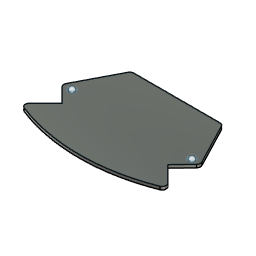
moter-size (Autodesk Fusion 360 design; units mm, degrees)
Autodesk Fusion 360 part; units mm, degrees
sketch "スケッチ1" plane through (0, 0, 0) normal (0, 0, 1) x (1, 0, 0)
  arc A0 (-42.8671, 10.2928) -> (42.0947, 10.2928) centre (-0.3862, 91.8977) ccw
  line L0 (-0.3862, 91.8977) -> (-42.8671, 10.2928) construction
  line L1 (-0.3862, 91.8977) -> (42.0947, 10.2928) construction
  line L2 (-42.8671, 10.2928) -> (-23.0119, 48.4342)
  line L3 (42.0947, 10.2928) -> (22.2395, 48.4342)
  line L4 (-23.0119, 48.4342) -> (22.2395, 48.4342)
  dimension "d1" = 92
  dimension "d2" = 55
  dimension "d3" = 43
  dimension "d4" = 43
  constraint parallel L0 L2
  constraint parallel L1 L3
  measures "d1" radius of A0
  measures "d2" angle of L0 L1
  measures "d3" distance of A0.start L2.end
  measures "d4" distance of A0.end L3.end
extrude "押し出し1" add sketch "スケッチ1" along normal blind 1.5
sketch "スケッチ2" plane through (0, 0, 1.5) normal (0, 0, 1) x (-1, 0, 0)
  arc A0 (42.8671, -10.2928) -> (-42.0947, -10.2928) centre (0.3862, -91.8977) ccw
  line L0 (-42.0947, -10.2928) -> (-22.2395, -48.4342)
  line L1 (-22.2395, -48.4342) -> (23.0119, -48.4342)
  line L2 (23.0119, -48.4342) -> (42.8671, -10.2928)
  line L3 (42.8671, -10.2928) -> (34.7865, -25.8154)
  line L4 (-42.0947, -10.2928) -> (-34.0141, -25.8154)
  line L5 (34.7865, -25.8154) -> (26.6537, -17.6847)
  line L6 (26.6537, -17.6847) -> (36.8874, -7.4486)
  line L7 (36.8874, -7.4486) -> (42.8671, -10.2928)
  line L8 (34.7865, -25.8154) -> (42.8671, -10.2928)
  line L9 (-34.0141, -25.8154) -> (-26.0125, -17.5556)
  line L10 (-26.0125, -17.5556) -> (-36.1199, -7.4507)
  line L11 (-36.1199, -7.4507) -> (-42.0947, -10.2928)
  dimension "d7" = 17.5
  dimension "d8" = 17.5
  dimension "d9" = 11.5
  dimension "d10" = 11.5
  constraint coincident A0.start L2.end
  constraint parallel L2 L3
  constraint coincident A0.end L0.start
  constraint parallel L0 L4
  constraint coincident A0 L6.end
  constraint perpendicular L5 L6
  constraint coincident A0 L10.end
  constraint perpendicular L6 L10
  measures "d7" distance of A0.start L3.end
  measures "d8" distance of A0.end L4.end
  measures "d9" distance of L3.end L5.end
  measures "d10" distance of L4.end L9.end
extrude "押し出し2" cut sketch "スケッチ2" against normal blind 1.5 contours L2 L3 L5 L6 L7 L8
extrude "押し出し3" cut sketch "スケッチ2" against normal blind 1.5 contours L0 L4 L9 L10 L11
sketch "スケッチ3" plane through (0, 0, 1.5) normal (0, 0, 1) x (-1, 0, 0)
  line L0 (-36.1199, -7.4507) -> (-26.0125, -17.5556)
  line L1 (-26.0125, -17.5556) -> (-34.0141, -25.8154)
  line L2 (-34.0141, -25.8154) -> (-22.2395, -48.4342)
  line L3 (-22.2395, -48.4342) -> (23.0119, -48.4342)
  line L4 (23.0119, -48.4342) -> (34.7865, -25.8154)
  line L5 (34.7865, -25.8154) -> (26.6537, -17.6847)
  line L6 (26.6537, -17.6847) -> (36.8874, -7.4486)
  arc A0 (36.8874, -7.4486) -> (-36.1199, -7.4507) centre (0.3862, -91.8977) ccw
  line L7 (45.6832, -13.5395) -> (36.8874, -13.5395)
  line L8 (36.8874, -13.5395) -> (36.8874, -7.4486)
  line L9 (36.8874, -7.4486) -> (45.6832, -7.4486)
  line L10 (45.6832, -7.4486) -> (45.6832, -13.5395)
  line L11 (-36.1199, -7.4507) -> (-43.0096, -7.4507)
  line L12 (-43.0096, -7.4507) -> (-43.0096, -10.616)
  line L13 (-43.0096, -10.616) -> (-36.1199, -10.616)
  line L14 (-36.1199, -10.616) -> (-36.1199, -7.4507)
  constraint horizontal L7
  constraint vertical L8
  constraint horizontal L9
  constraint vertical L10
  constraint coincident L6.end A0.start
  constraint horizontal L11
  constraint vertical L12
  constraint horizontal L13
  constraint vertical L14
  constraint coincident L0.start A0.end
extrude "押し出し4" cut sketch "スケッチ3" against normal blind 1.5 contours L7 L8 L9 L10
extrude "押し出し5" cut sketch "スケッチ3" against normal blind 1.5 contours L11 L12 L13 L14
fillet "フィレット1" radius 2 1 edges at (-36.8874, 7.4486, 0.75)
fillet "フィレット2" radius 2 1 edges at (-34.7865, 25.8154, 0.75)
fillet "フィレット3" radius 2 1 edges at (36.1199, 7.4507, 0.75)
fillet "フィレット4" radius 2 1 edges at (22.2395, 48.4342, 0.75)
fillet "フィレット5" radius 2 1 edges at (-23.0119, 48.4342, 0.75)
fillet "フィレット6" radius 2 1 edges at (34.0141, 25.8154, 0.75)
sketch "スケッチ4" plane through (0, 0, 1.5) normal (0, 0, 1) x (-1, 0, 0)
  arc A0 (-33.0106, -24.7796) -> (-33.3482, -27.0947) centre (-31.5741, -26.1712) ccw
  line L0 (-33.3482, -27.0947) -> (-22.7999, -47.3577)
  arc A1 (-22.7999, -47.3577) -> (-21.0259, -48.4342) centre (-21.0259, -46.4342) ccw
  line L1 (-21.0259, -48.4342) -> (21.7982, -48.4342)
  arc A2 (21.7982, -48.4342) -> (23.5723, -47.3577) centre (21.7982, -46.4342) ccw
  line L2 (23.5723, -47.3577) -> (34.1092, -27.1164)
  arc A3 (34.1092, -27.1164) -> (33.7492, -24.7785) centre (32.3352, -26.1929) ccw
  line L3 (33.7492, -24.7785) -> (26.6537, -17.6847)
  line L4 (26.6537, -17.6847) -> (34.7689, -9.5676)
  arc A4 (34.7689, -9.5676) -> (34.0871, -6.2926) centre (33.3545, -8.1536) ccw
  arc A5 (34.0871, -6.2926) -> (-33.3191, -6.2943) centre (0.3862, -91.8977) ccw
  arc A6 (-33.3191, -6.2943) -> (-34.0004, -9.5696) centre (-32.5864, -8.1552) ccw
  line L5 (-34.0004, -9.5696) -> (-26.0125, -17.5556)
  line L6 (-26.0125, -17.5556) -> (-33.0106, -24.7796)
  circle A7 centre (30, -26) radius 1.5
  circle A8 centre (-29.6492, -25.8885) radius 1.5
  dimension "d31" = 3
  dimension "d32" = 3
  measures "d31" diameter of A7
  measures "d32" diameter of A8
extrude "押し出し6" cut sketch "スケッチ4" against normal blind 2 contours A8
extrude "押し出し7" cut sketch "スケッチ4" against normal blind 2 contours A7
